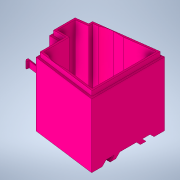
# Autodesk Inventor part: hull_electronics
Saved by Autodesk Inventor 2020 (Build 240168000, 168)
## iProperties
Created: 2019-09-19
Part Number: hull_electronics
Material: Generic
Document SubType Name: Modeling
Designer: suchanek
Density: 1 g/cm^3
Appearance: Default
Author: suchanek
Autodesk Inventor part; units mm, degrees
ref_plane "YZ Plane" through (0, 0, 0) normal (1, 0, 0) x (0, 1, 0)
ref_plane "XZ Plane" through (0, 0, 0) normal (0, 1, 0) x (-1, 0, 0)
sketch "Sketch1" plane through (0, 0, 0) normal (0, 0, 1) x (1, 0, 0)
  arc A0 (-28, 102.5) -> (-17, 102.5) centre (-22.5, 102.5) ccw projected
  line L0 (-17, 102.5) -> (0, 102.5) projected
  line L1 (0, 102.5) -> (0, 130) projected
  line L2 (0, 130) -> (5, 130) projected
  line L3 (5, 130) -> (10, 92.0212) projected
  line L4 (10, 92.0212) -> (10, 30) projected
  line L5 (10, 30) -> (23.1652, -70) projected
  line L6 (23.1652, -70) -> (-68.1652, -70) projected
  line L7 (-68.1652, -70) -> (-55, 30) projected
  line L8 (-55, 30) -> (-55, 92.0212) projected
  line L9 (-55, 92.0212) -> (-50, 130) projected
  line L10 (-50, 130) -> (-45, 130) projected
  line L11 (-45, 130) -> (-45, 102.5) projected
  line L12 (-45, 102.5) -> (-28, 102.5) projected
  line L13 (-60.2661, -10) -> (15.2661, -10) projected
  line L14 (15.2661, -10) -> (12.633, 10) projected
  line L15 (7.5899, 10) -> (12.633, 10) projected
  line L16 (5.6151, 25) -> (7.5899, 10) projected
  line L17 (-50.6151, 25) -> (5.6151, 25) projected
  line L18 (-52.5899, 10) -> (-50.6151, 25) projected
  line L19 (-57.633, 10) -> (-52.5899, 10) projected
  line L20 (-57.633, 10) -> (-60.2661, -10) projected
  line L21 (-26, 25) -> (-26, 30) projected
  line L22 (-26, 25) -> (-26, 10)
  line L23 (-26, 10) -> (-57.633, 10)
  line L24 (-57.633, 10) -> (-68.1652, -70)
  line L25 (23.1652, -70) -> (-68.1652, -70)
  line L26 (23.1652, -70) -> (12.633, 10)
  line L27 (12.633, 10) -> (7.5899, 10)
  line L28 (7.5899, 10) -> (5.6151, 25)
  line L29 (-26, 25) -> (5.6151, 25)
  point P0 (0, 0)
  constraints: 16 end point, 2 collinear, 2 parallel, 1 horizontal, 1 point on line, 1 vertical
extrude "Extrusion1" add sketch "Sketch1" along normal blind 5 and the other way blind 5 contours L19 L23 L22 L17 L16 L15 L5 L13 L7 | L13 L5 L6 L7
sketch "Sketch3" plane through (-68.1652, -70, 5) normal (0, -1, 0) x (1, 0, 0)
  line L0 (0, -25) -> (0, -10)
  line L1 (0, -10) -> (91.3305, -10)
  line L2 (91.3305, -10) -> (91.3305, -25)
  line L3 (91.3305, -25) -> (0, -25)
  line L4 (28.1652, -5) -> (23.1652, -10)
  line L5 (23.1652, -10) -> (13.1652, -10)
  line L6 (13.1652, -10) -> (18.1652, -5)
  line L7 (18.1652, -5) -> (28.1652, -5)
  line L8 (68.1652, -10) -> (63.1652, -5)
  line L9 (63.1652, -5) -> (73.1652, -5)
  line L10 (73.1652, -5) -> (78.1652, -10)
  line L11 (78.1652, -10) -> (68.1652, -10)
  line L12 (10.5322, -10) -> (42.1652, -10) projected
  line L13 (30.2363, -10) -> (35.2363, -5)
  line L14 (35.2363, -5) -> (56.0942, -5)
  line L15 (56.0942, -5) -> (61.0942, -10)
  line L16 (42.1652, -10) -> (73.7804, -10) projected
  line L17 (30.2363, -10) -> (61.0942, -10)
  point P0 (68.1652, -5)
  dimension "d6" = 5
  dimension "d7" = 5
  constraints: 30 end point, 6 horizontal, 3 parallel, 2 point on line, 2 vertical, 1 collinear, 19 other
  measures "d6" distance between parallel lines of L13 L4
  measures "d7" distance between parallel lines of L8 L15
extrude "Extrusion2" cut sketch "Sketch3" against normal through all contours L6 L7 L4 L1 | L1 L8 L9 L10 | L13 L14 L15 L1
sketch "Sketch4" plane through (0, 0, 5) normal (0, 0, 1) x (1, 0, 0)
  line L0 (7.5899, 10) -> (5.6151, 25) projected
  line L1 (5.6151, 25) -> (-26, 25) projected
  line L2 (-26, 25) -> (-26, 10) projected
  line L3 (-26, 10) -> (-57.633, 10) projected
  line L4 (-57.633, 10) -> (-68.1652, -70) projected
  line L5 (-68.1652, -70) -> (23.1652, -70) projected
  line L6 (23.1652, -70) -> (12.633, 10) projected
  line L7 (12.633, 10) -> (7.5899, 10) projected
  line L8 (-62.4638, -65) -> (-53.2482, 5)
  line L9 (-53.2482, 5) -> (-21, 5)
  line L10 (-21, 5) -> (-21, 20)
  line L11 (-21, 20) -> (1.2302, 20)
  line L12 (1.2302, 20) -> (3.205, 5)
  line L13 (3.205, 5) -> (8.2482, 5)
  line L14 (10, -70) -> (10, 10) projected
  line L15 (8.2482, 5) -> (17.4638, -65)
  line L16 (17.4638, -65) -> (-62.4638, -65)
  line L17 (-26, 10) -> (-57.633, 10) projected
  line L18 (5.6151, 25) -> (-26, 25) projected
  line L19 (7.5899, 10) -> (5.6151, 25) projected
  line L20 (12.633, 10) -> (7.5899, 10) projected
  line L21 (-68.1652, -70) -> (23.1652, -70) projected
  point P0 (0, 0)
  dimension "d8" = 5
  dimension "d9" = 5
  dimension "d10" = 5
  dimension "d11" = 5
  dimension "d12" = 5
  dimension "d13" = 5
  dimension "d14" = 5
  dimension "d15" = 5
  constraints: 16 end point, 10 parallel, 3 perpendicular
  measures "d8" distance between parallel lines of L4 L8
  measures "d9" distance between parallel lines of L3 L9
  measures "d10" distance between parallel lines of L2 L10
  measures "d11" distance between parallel lines of L1 L11
  measures "d12" distance between parallel lines of L0 L12
  measures "d13" distance between parallel lines of L20 L13
  measures "d14" distance between parallel lines of L6 L15
  measures "d15" distance between parallel lines of L5 L16
extrude "Extrusion3" add sketch "Sketch4" along normal blind 70 contours L7 L14 L15 L13 L12 L11 L10 L9 L8 L16 L5 L4 L3 L2 L1 L0 | L7 L6 L5 L14 L16 L15
sketch "Sketch5" plane through (0, 0, 75) normal (0, 0, 1) x (1, 0, 0)
  line L0 (-65.1435, -67.35) -> (-55.3091, 7.35)
  line L1 (-68.1652, -70) -> (-57.633, 10) projected
  line L2 (-55.3091, 7.35) -> (-23.35, 7.35)
  line L3 (-23.35, 7.35) -> (-23.35, 22.35)
  line L4 (-23.35, 22.35) -> (3.4424, 22.35)
  line L5 (3.4424, 22.35) -> (5.4172, 7.35)
  line L6 (5.4172, 7.35) -> (10.3091, 7.35)
  line L7 (10.3091, 7.35) -> (20.1435, -67.35)
  line L8 (20.1435, -67.35) -> (-65.1435, -67.35)
  line L9 (-62.4638, -65) -> (-53.2482, 5) projected
  line L10 (-53.2482, 5) -> (-21, 5) projected
  line L11 (-21, 5) -> (-21, 20) projected
  line L12 (-21, 20) -> (1.2302, 20) projected
  line L13 (1.2302, 20) -> (3.205, 5) projected
  line L14 (3.205, 5) -> (8.2482, 5) projected
  line L15 (8.2482, 5) -> (17.4638, -65) projected
  line L16 (17.4638, -65) -> (-62.4638, -65) projected
  point P0 (0, 0)
  dimension "d19" = 2.35
  dimension "d20" = 2.35
  dimension "d21" = 2.35
  dimension "d22" = 2.5
  dimension "d23" = 2.35
  dimension "d24" = 2.35
  dimension "d25" = 2.35
  constraints: 16 end point, 10 parallel, 2 perpendicular, 2 point on line, 1 horizontal
  measures "d19" distance between parallel lines of L16 L8
  measures "d20" distance between parallel lines of L7 L15
  measures "d21" distance between parallel lines of L6 L14
  measures "d22" distance between parallel lines of L5 L13
  measures "d23" distance between parallel lines of L4 L12
  measures "d24" distance between parallel lines of L11 L3
  measures "d25" distance between parallel lines of L0 L9
extrude "Extrusion4" add sketch "Sketch5" along normal blind 6
sketch "Sketch6" plane through (7.5899, 10, 75) normal (0.9914449, 0.1305262, 0) x (0, 0, -1)
  line L0 (75.6151, 15.1294) -> (0, 15.1294) projected
  line L1 (77.5899, 0) -> (0, 0) projected
  line L2 (10.6151, 25.1294) -> (20.6151, 25.1294)
  line L3 (20.6151, 25.1294) -> (20.6151, 0)
  line L4 (20.6151, 0) -> (10.6151, 0)
  line L5 (10.6151, 0) -> (10.6151, 25.1294)
  point P0 (75, -8.9238)
  point P1 (10.6151, 0)
  point P2 (20.6151, 15.1294)
  point P3 (10.6151, 15.1294)
  dimension "d29" = 10
  dimension "d30" = 55
  dimension "d33" = 10
  constraints: 8 end point, 2 parallel, 1 horizontal, 1 perpendicular, 1 point on line
  measures "d29" distance of L3.end L4.end
  measures "d30" distance from line of L3 L0.start
  measures "d33" distance between parallel lines of L0 L2
extrude "Extrusion5" cut sketch "Sketch6" against normal blind 4
sketch "Sketch7" plane through (7.5899, 10, 64.3849) normal (-0.1305262, 0.9914449, 0) x (0.9914449, 0.1305262, 0)
  line L0 (1.8, 9) -> (3, 9)
  line L1 (3, 9) -> (3, 1)
  line L2 (3, 1) -> (1.8, 1)
  line L3 (1.8, 1) -> (1.8, 9)
  line L4 (0, 10) -> (0, 0) projected
  line L5 (-4, 10) -> (0, 10) projected
  line L6 (0, 0) -> (-4, 0) projected
  line L7 (-4, 0) -> (-4, 10) projected
  point P0 (-8.8302, 64.3849)
  dimension "d34" = 1.2
  dimension "d37" = 1
  dimension "d38" = 1
  dimension "d49" = 5.8
  constraints: 8 end point, 2 parallel, 1 horizontal, 1 perpendicular
  measures "d34" distance of L1.end L2.end
  measures "d37" distance between parallel lines of L5 L0
  measures "d38" distance between parallel lines of L6 L2
  measures "d49" distance between parallel lines of L7 L3
extrude "Extrusion6" add sketch "Sketch7" along normal blind 15 and the other way blind 2 contours L0 L1 L2 L3
sketch "Sketch8" plane through (10.6158, 10, 63.3849) normal (0.9914449, 0.1305262, 0) x (0, 0, -1)
  line L0 (0, 15.395) -> (8, 15.395) projected
  line L1 (8, 0) -> (8, 15.395) projected
  line L2 (0, 15.395) -> (8, 15.395)
  line L3 (8, 15.395) -> (8, 12.395)
  line L4 (8, 12.395) -> (0, 12.395)
  line L5 (0, 12.395) -> (0, 15.395)
  point P0 (63.3849, -8.5288)
  dimension "d43" = 3
  constraints: 8 end point, 2 parallel, 1 horizontal, 1 perpendicular, 1 point on line
  measures "d43" distance of L4.end L0.start
extrude "Extrusion7" add sketch "Sketch8" along normal blind 3
chamfer "Chamfer1" distance 2 angle 45 1 edges at (11.5807, 25.6548, 59.3849)
ref_plane "Work Plane1" through (-22.5, 276.862, -5) normal (-1, 0, 0) x (0, 0, 1)
mirror "Mirror1" about plane through (-22.5, 276.862, -5) normal (-1, 0, 0) of "Extrusion7", "Extrusion6", "Chamfer1"
sketch "Sketch9" plane through (-26, 25, 0) normal (0, 1, 0) x (1, 0, 0)
  line L0 (-42.1652, 0) -> (49.1652, 0)
  line L1 (49.1652, 0) -> (49.1652, 5)
  line L2 (49.1652, 5) -> (-42.1652, 5)
  line L3 (-42.1652, 5) -> (-42.1652, 0)
  line L4 (49.1652, 5) -> (49.1652, -75) projected
  line L5 (38.633, 5) -> (49.1652, 5) projected
  line L6 (-42.1652, 5) -> (-42.1652, -75) projected
  line L7 (31, 0) -> (21, 0) projected
  point P0 (26, 0)
  constraints: 8 end point, 4 collinear, 2 parallel, 1 horizontal, 1 perpendicular
extrude "Extrusion8" cut sketch "Sketch9" against normal up to surface (15 mm away)
sketch "Sketch10" plane through (0, 0, 81) normal (0, 0, 1) x (1, 0, 0)
  line L0 (-53.2482, 5) -> (-62.4638, -65) projected
  arc A0 (-54.1259, -1.6671) -> (-56.9375, -23.0235) centre (-27.7713, -16) ccw
  line L1 (8.2482, 5) -> (17.4638, -65) projected
  arc A1 (11.9375, -23.0235) -> (9.1259, -1.6671) centre (-17.2287, -16) ccw
  line L2 (-62.4638, -65) -> (-53.2482, 5) projected
  line L3 (-56.6411, -5.4489) -> (-58.5479, -19.9328)
  line L4 (-57.633, 10) -> (-68.1652, -70) projected
  line L5 (-57.7713, -16) -> (-57.7713, -29.3563)
  line L6 (12.7713, -16) -> (12.7713, -29.3563)
  line L7 (17.4638, -65) -> (-62.4638, -65) projected
  point P0 (0, 0)
  point P1 (-57.7713, -29.3563)
  dimension "d52" = 3
  dimension "d54" = 30
  dimension "d57" = 49
  constraints: 6 end point, 6 point on circle, 6 point on line, 3 tangent, 2 centre point, 2 horizontal alignment, 2 vertical, 1 equal radius, 1 parallel
  measures "d52" distance between parallel lines of L4 L3
  measures "d54" radius of A0
  measures "d57" distance from line of L7 A0.centre
extrude "Extrusion9" cut sketch "Sketch10" against normal up to surface (76 mm away)
equation "\"d19\" = d25"
equation "\"d20\" = d25"
equation "\"d21\" = d25"
equation "\"d23\" = d25"
equation "\"d24\" = d25"
body "Solid1"
